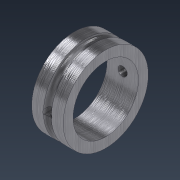
# Autodesk Inventor part: Łożysko wału korbowego
Saved by Autodesk Inventor 2022 (Build 260153000, 153)
## iProperties
Created: 2023-05-20
Part Number: Łożysko wału korbowego
Material: Generic
Document SubType Name: Modeling
Designer: wikto
Density: 1 g/cm^3
Appearance: Machined 03
Mass: 29.341 g
Surface Area: 120.484 cm^2
Volume: 29.341 cm^3
Author: wikto
Autodesk Inventor part; units mm, degrees
ref_plane "YZ Plane" through (0, 0, 0) normal (1, 0, 0) x (0, 1, 0)
ref_plane "XZ Plane" through (0, 0, 0) normal (0, 1, 0) x (-1, 0, 0)
ref_plane "XY Plane" through (0, 0, 0) normal (0, 0, 1) x (1, 0, 0)
sketch "Sketch1" plane through (0, 0, 0) normal (0, 1, 0) x (-1, 0, 0)
  line L0 (100, 0) -> (-100, 0)
  line L1 (12, -25) -> (12, -32.5)
  line L2 (12, -32.5) -> (3, -32.5)
  line L3 (-3, -32.5) -> (-12, -32.5)
  line L4 (-12, -32.5) -> (-12, -25)
  arc A0 (3, -32.5) -> (-3, -32.5) centre (0, -32.5) ccw
  line L5 (12, -25) -> (-12, -25)
  point P0 (0, 0)
  point P1 (0, 0)
  dimension "d0" = 200
  dimension "d1" = 65
  dimension "d2" = 24
  dimension "d3" = 3
  dimension "d5" = 50
  constraints: 12 end point, 3 horizontal, 2 horizontal alignment, 2 perpendicular, 2 point on circle, 1 centre point, 1 coincident, 1 collinear, 1 midpoint, 1 vertical, 1 vertical alignment
  measures "d0" distance of L0.start L0.end
  measures "d1" diameter of L3 L0
  measures "d2" distance between parallel lines of L1 L4
  measures "d3" radius of A0
  measures "d5" diameter of L5 L0
revolve "Revolution1" add sketch "Sketch1" angle 360 about axis through (-100, 0, 0) along (1, 0, 0)
sketch "Sketch2" plane through (0, 0, 0) normal (0, 0, 1) x (1, 0, 0)
  circle A0 centre (0, 0) radius 3.5
  dimension "d6" = 7
  constraints: 1 centre point, 1 coincident
  measures "d6" diameter of A0
extrude "Extrusion1" cut sketch "Sketch2" along normal through all both and the other way through all
body "Solid1"
